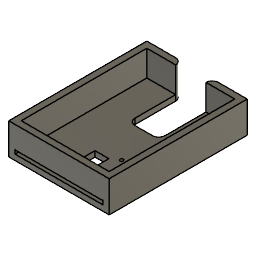
Upper_Card_Holder (Autodesk Fusion 360 design; units mm, degrees)
Autodesk Fusion 360 part; units mm, degrees
sketch "Çizim1" plane through (0, 0, 0) normal (0, 0, 1) x (1, 0, 0)
  line L0 (35, 50) -> (-35, 50)
  line L1 (-35, 50) -> (-35, -50)
  line L2 (-35, -50) -> (35, -50)
  line L3 (35, -50) -> (35, 50)
  line L4 (35, 50) -> (-35, -50) construction
  line L5 (-35, 50) -> (35, -50) construction
  line L6 (-40, -55) -> (40, -55)
  line L7 (40, -55) -> (40, 55)
  line L8 (40, 55) -> (-40, 55)
  line L9 (-40, 55) -> (-40, -55)
  dimension "d1" = 70
  dimension "d2" = 100
  dimension "d3" = 5
  constraint horizontal L0
  constraint perpendicular L0 L1
  constraint parallel L0 L2
  constraint parallel L1 L3
  constraint coincident L4 origin
  constraint coincident L5 origin
  measures "d1" distance of L1.end L2.end
  measures "d2" distance of L0.end L1.end
extrude "Ekstrüzyon1" add sketch "Çizim1" against normal blind 5 contours L0 L1 L2 L3 | L6 L7 L8 L9
extrude "Ekstrüzyon2" add sketch "Çizim1" along normal blind 20
sketch "Çizim2" plane through (0, -50, 0) normal (0, 1, 0) x (-1, 0, 0)
  line L0 (-35, 0) -> (35, 0)
  line L1 (35, 0) -> (35, 20)
  line L2 (35, 20) -> (-35, 20)
  line L3 (-35, 20) -> (-35, 0)
  line L4 (-35, 0) -> (35, 0)
  line L5 (35, 0) -> (35, 2.4)
  line L6 (35, 2.4) -> (-35, 2.4)
  line L7 (-35, 2.4) -> (-35, 0)
  dimension "d8" = 2.4
  constraint horizontal L4
  constraint vertical L5
  constraint horizontal L6
  constraint vertical L7
  constraint coincident L0.start L3.end
  measures "d8" distance of L0.start L6.end
extrude "Ekstrüzyon3" cut sketch "Çizim2" against normal blind 5 contours L0 L1 L3 L4 L5 L6 L7
sketch "Çizim3" plane through (0, 0, 20) normal (0, 0, 1) x (-1, 0, 0)
  line L0 (-35, -50) -> (-35, 50)
  line L1 (-35, 50) -> (35, 50)
  line L2 (35, 50) -> (35, -50)
  line L3 (35, -50) -> (-35, -50)
  line L4 (40, -55) -> (40, 55)
  line L5 (40, 55) -> (-40, 55)
  line L6 (-40, 55) -> (-40, -55)
  line L7 (-40, -55) -> (40, -55)
  line L8 (12, -12.5) -> (-12, -12.5)
  line L9 (-12, -12.5) -> (-12, -87.5)
  line L10 (-12, -87.5) -> (12, -87.5)
  line L11 (12, -87.5) -> (12, -12.5)
  line L12 (12, -12.5) -> (-12, -87.5) construction
  line L13 (-12, -12.5) -> (12, -87.5) construction
  point P0 (0, -50)
  dimension "d11" = 75
  constraint horizontal L8
  constraint perpendicular L8 L9
  constraint parallel L8 L10
  constraint parallel L9 L11
  constraint coincident L12 P0
  constraint coincident L13 P0
  constraint midpoint L3 P0
  measures "d11" distance of L8.end L9.end
extrude "Ekstrüzyon4" cut sketch "Çizim3" against normal blind 25 contours L3 L8 L9 L11 | L3 L7 L9 L11
fillet "Radyus1" radius 5 4 edges at (12, 55, 7.5) (-12, 55, 7.5) (12, 12.5, -2.5) (-12, 12.5, -2.5)
chamfer "Pah1" distance 5 angle 45 1 edges at (0, -50, 2.4) tangent chain off
sketch "Çizim4" plane through (0, 0, -5) normal (0, 0, -1) x (1, 0, 0)
  arc A0 (-17, -55) -> (-12, -50) centre (-17, -50) ccw
  line L0 (-12, -50) -> (-12, -17.5)
  arc A1 (-7, -12.5) -> (-12, -17.5) centre (-7, -17.5) ccw
  line L1 (-7, -12.5) -> (7, -12.5)
  arc A2 (12, -17.5) -> (7, -12.5) centre (7, -17.5) ccw
  line L2 (12, -17.5) -> (12, -50)
  arc A3 (12, -50) -> (17, -55) centre (17, -50) ccw
  line L3 (17, -55) -> (40, -55)
  line L4 (40, -55) -> (40, 55)
  line L5 (40, 55) -> (-40, 55)
  line L6 (-40, 55) -> (-40, -55)
  line L7 (-40, -55) -> (-17, -55)
  line L8 (0, 55) -> (0, 11.6)
  line L9 (0, 11.6) -> (0, 30.8)
  line L10 (-4.5, 25.8) -> (4.5, 25.8)
  line L11 (4.5, 25.8) -> (4.5, 35.8)
  line L12 (4.5, 35.8) -> (-4.5, 35.8)
  line L13 (-4.5, 35.8) -> (-4.5, 25.8)
  line L14 (-4.5, 25.8) -> (4.5, 35.8) construction
  line L15 (4.5, 25.8) -> (-4.5, 35.8) construction
  point P0 (0, 30.8)
  dimension "d17" = 43.4
  dimension "d18" = 19.2
  dimension "d19" = 9
  dimension "d20" = 10
  constraint midpoint L5 L8.start
  constraint perpendicular L5 L8
  constraint parallel L8 L9
  constraint horizontal L10
  constraint perpendicular L10 L11
  constraint parallel L10 L12
  constraint parallel L11 L13
  constraint coincident L14 P0
  constraint coincident L15 P0
  constraint coincident P0 L9.end
  measures "d17" distance of L8.start L8.end
  measures "d18" distance of L8.end P0
  measures "d19" distance of L11.end L12.end
  measures "d20" distance of L10.end L11.end
extrude "Ekstrüzyon5" cut sketch "Çizim4" against normal blind 5 contours L8 L9 L10 L11 L12 | L8 L9 L10 L12 L13
sketch "Çizim5" plane through (0, 0, 0) normal (0, 0, 1) x (-1, 0, 0)
  line L0 (4.5, 25.8) -> (-4.5, 25.8)
  line L1 (-4.5, 25.8) -> (-4.5, 35.8)
  line L2 (-4.5, 35.8) -> (4.5, 35.8)
  line L3 (4.5, 35.8) -> (4.5, 25.8)
  line L4 (12, -17.5) -> (12, -50)
  line L5 (12, -50) -> (35, -50)
  line L6 (35, -50) -> (35, 55)
  line L7 (35, 55) -> (-35, 55)
  line L8 (-35, 55) -> (-35, -50)
  line L9 (-35, -50) -> (-12, -50)
  line L10 (-12, -50) -> (-12, -17.5)
  arc A0 (-7, -12.5) -> (-12, -17.5) centre (-7, -17.5) ccw
  line L11 (-7, -12.5) -> (7, -12.5)
  arc A1 (12, -17.5) -> (7, -12.5) centre (7, -17.5) ccw
  line L12 (-11.6, 30.8) -> (-29.1, 30.8)
  line L13 (-11.6, 30.8) -> (-11.6, 16.6)
  line L14 (-11.6, 30.8) -> (-11.6, 45)
  circle A2 centre (-11.6, 45) radius 1.3
  circle A3 centre (-11.6, 16.6) radius 1.3
  circle A4 centre (-11.6, 16.6) radius 3
  circle A5 centre (-11.6, 45) radius 3
  dimension "d23" = 14.2
  dimension "d24" = 14.2
  dimension "d25" = 2.6
  dimension "d26" = 2.6
  dimension "d27" = 6
  dimension "d28" = 6
  dimension "d43" = 9.2
  dimension "d44" = 16.1
  constraint perpendicular L0 L13
  constraint coincident L14.end A2.centre
  constraint coincident L13.end A3.centre
  constraint concentric A3 A4
  constraint concentric A2 A5
  measures "d23" distance of L12.start L13.end
  measures "d24" distance of L12.start L14.end
  measures "d25" diameter of A2
  measures "d26" diameter of A3
  measures "d27" diameter of A4
  measures "d28" diameter of A5
  measures "d43" distance of L2 L14.end
  measures "d44" distance of L3 L14.end
extrude "Ekstrüzyon6" cut sketch "Çizim5" against normal blind 3 contours A2 | A3 | A4 | A5
extrude "Ekstrüzyon7" cut sketch "Çizim5" against normal blind 5 contours A2 | A3
extrude "Ekstrüzyon8" cut 1 faces at (-27.2658, 3.6971, 0) along direction (0, 0, -1) blind 0.5
extrude "Ekstrüzyon9" cut 1 faces at (-4.5, -32.4667, -3.5) along direction (-1, 0, 0) blind 1
extrude "Ekstrüzyon10" cut 1 faces at (1.1667, -35.8, -3.5) along direction (0, -1, 0) blind 1
extrude "Ekstrüzyon11" cut 1 faces at (-2.1667, -25.8, -2) along direction (0, 1, 0) blind 1
extrude "Ekstrüzyon12" cut 1 faces at (4.5, -32.8, -3.5) along direction (1, 0, 0) blind 1
sketch "Çizim6" plane through (0, 0, -0.5) normal (0, 0, 1) x (-1, 0, 0)
  circle A0 centre (-11.6, 16.6) radius 3
  circle A1 centre (-11.6, 45) radius 3
  line L0 (5.5, 24.8) -> (-5.5, 24.8)
  line L1 (-5.5, 24.8) -> (-5.5, 36.8)
  line L2 (-5.5, 36.8) -> (5.5, 36.8)
  line L3 (5.5, 36.8) -> (5.5, 24.8)
  line L4 (12, -17.5) -> (12, -50)
  line L5 (12, -50) -> (35, -50)
  line L6 (35, -50) -> (35, 55)
  line L7 (35, 55) -> (-35, 55)
  line L8 (-35, 55) -> (-35, -50)
  line L9 (-35, -50) -> (-12, -50)
  line L10 (-12, -50) -> (-12, -17.5)
  arc A2 (-7, -12.5) -> (-12, -17.5) centre (-7, -17.5) ccw
  line L11 (-7, -12.5) -> (7, -12.5)
  arc A3 (12, -17.5) -> (7, -12.5) centre (7, -17.5) ccw
  line L12 (-5.5, 24.8) -> (5.5, 24.8)
  line L13 (5.5, 24.8) -> (5.5, 36.8)
  line L14 (5.5, 36.8) -> (-5.5, 36.8)
  line L15 (-5.5, 36.8) -> (-5.5, 24.8)
  line L16 (-5.5, 36.8) -> (5.5, 36.8)
  line L17 (5.5, 36.8) -> (5.5, 40.8)
  line L18 (5.5, 40.8) -> (-5.5, 40.8)
  line L19 (-5.5, 40.8) -> (-5.5, 36.8)
  line L20 (-5.5, 24.8) -> (5.5, 24.8)
  line L21 (5.5, 24.8) -> (5.5, 20.8)
  line L22 (5.5, 20.8) -> (-5.5, 20.8)
  line L23 (-5.5, 20.8) -> (-5.5, 24.8)
  dimension "d45" = 4
  dimension "d46" = 11
  dimension "d47" = 4
  constraint horizontal L12
  constraint vertical L13
  constraint horizontal L14
  constraint vertical L15
  constraint coincident L2.end L3.start
  constraint coincident L0.end L1.start
  constraint horizontal L16
  constraint vertical L17
  constraint horizontal L18
  constraint vertical L19
  constraint coincident L1.end L2.start
  constraint horizontal L20
  constraint vertical L21
  constraint horizontal L22
  constraint vertical L23
  measures "d45" distance of L1.end L18.end
  measures "d46" distance of L0.end L0.start
  measures "d47" distance of L0.end L22.end
extrude "Ekstrüzyon13" cut sketch "Çizim6" against normal blind 4.5 contours L0 L12 L20 L21 L22 L23 | L2 L14 L16 L17 L18 L19
extrude "Ekstrüzyon14" add 2 faces at (9.1827, -16.3864, -3) (14.0173, -44.7864, -3) along direction (0, 0, 1) blind 2.5
equation "d17 = 38.40 mm + 5 mm"
equation "d23 = 6 mm + 13.20 mm - 5 mm"
equation "d24 = 6 mm + 13.20 mm - 5 mm"
equation "d44 = 9 mm + 7.1 mm"
